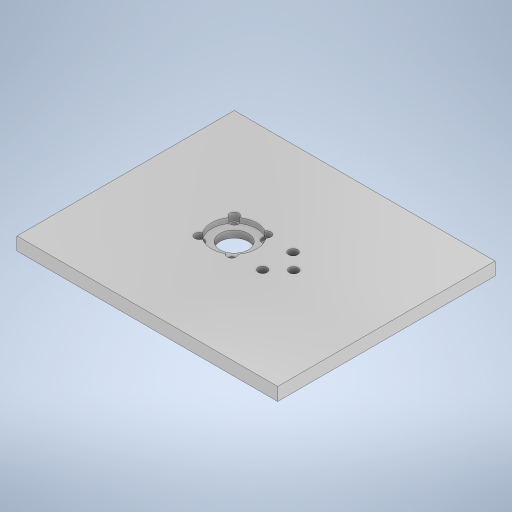
# Autodesk Inventor part: axis_1_top_frame
Saved by Autodesk Inventor 2024.1 (Build 281209000, 209)
## iProperties
Created: 2023-08-26
Part Number: axis_1_top_frame
Material: Aluminum 6061-AHC
Document SubType Name: Modeling
Designer: chanh
Density: 2.7 g/cm^3
Appearance: Aluminum - Dark
Author: chanh
Autodesk Inventor part; units mm, degrees
ref_plane "YZ Plane" through (0, 0, 0) normal (1, 0, 0) x (0, 1, 0)
ref_plane "XZ Plane" through (0, 0, 0) normal (0, 1, 0) x (-1, 0, 0)
ref_plane "XY Plane" through (0, 0, 0) normal (0, 0, 1) x (1, 0, 0)
sketch "Sketch1" plane through (0, 0, 0) normal (0, 1, 0) x (-1, 0, 0)
  line L0 (60, 50) -> (-60, 50)
  line L1 (-60, 50) -> (-60, -50)
  line L2 (-60, -50) -> (60, -50)
  line L3 (60, -50) -> (60, 50)
  line L4 (60, 50) -> (-60, -50) construction
  line L5 (-60, 50) -> (60, -50) construction
  point P0 (0, 0)
  dimension "d0" = 120
  dimension "d1" = 100
  constraints: 12 end point, 2 midpoint, 2 parallel, 1 horizontal, 1 perpendicular
  measures "d0" distance of L2.end L1.end
  measures "d1" distance of L1.end L0.end
extrude "Extrusion1" add sketch "Sketch1" along normal blind 6
sketch "Sketch3" plane through (0, 0, 0) normal (0, -1, 0) x (1, 0, 0)
  circle A0 centre (17.37, 0) radius 0.7835 projected
  circle A1 centre (10.07, 7) radius 0.7835 projected
  circle A2 centre (10.07, -7) radius 0.7835 projected
  circle A3 centre (-3.15, 8) radius 0.7835 projected
  circle A4 centre (-3.15, -8) radius 0.7835 projected
  line L0 (18.77, -6.07) -> (18.77, 6.07) projected
  line L1 (18.77, -6.07) -> (18.05, -6.07) projected
  arc A5 (18.05, -6.07) -> (16.05, -8.07) centre (18.05, -8.07) ccw projected
  line L2 (16.05, -8.07) -> (16.05, -8.79) projected
  line L3 (-16.05, -8.79) -> (16.05, -8.79) projected
  line L4 (-16.05, -8.79) -> (-16.05, -8.07) projected
  arc A6 (-16.05, -8.07) -> (-18.05, -6.07) centre (-18.05, -8.07) ccw projected
  line L5 (-18.05, -6.07) -> (-18.77, -6.07) projected
  line L6 (-18.77, 6.07) -> (-18.77, -6.07) projected
  line L7 (-18.77, 6.07) -> (-18.05, 6.07) projected
  arc A7 (-18.05, 6.07) -> (-16.05, 8.07) centre (-18.05, 8.07) ccw projected
  line L8 (-16.05, 8.07) -> (-16.05, 8.79) projected
  line L9 (16.05, 8.79) -> (-16.05, 8.79) projected
  line L10 (16.05, 8.79) -> (16.05, 8.07) projected
  arc A8 (16.05, 8.07) -> (18.05, 6.07) centre (18.05, 8.07) ccw projected
  line L11 (18.05, 6.07) -> (18.77, 6.07) projected
  circle A9 centre (-10.05, 0) radius 6.4 projected
  line L12 (19.09, 6.07) -> (19.09, -6.07)
  line L13 (16.05, -9.11) -> (-16.05, -9.11)
  line L14 (-19.09, -6.07) -> (-19.09, 6.07)
  line L15 (-16.05, 9.11) -> (16.05, 9.11)
  line L16 (16.05, 8.79) -> (16.05, 9.11)
  line L17 (18.77, 6.07) -> (19.09, 6.07)
  line L18 (18.77, -6.07) -> (19.09, -6.07)
  line L19 (16.05, -8.79) -> (16.05, -9.11)
  line L20 (-16.05, -8.79) -> (-16.05, -9.11)
  line L21 (-18.77, -6.07) -> (-19.09, -6.07)
  line L22 (-18.77, 6.07) -> (-19.09, 6.07)
  line L23 (-16.05, 8.79) -> (-16.05, 9.11)
  line L24 (16.15, 8.79) -> (16.15, 9.21)
  line L25 (16.15, 9.21) -> (-16.15, 9.21)
  line L26 (-16.15, 9.21) -> (-16.15, 8.79)
  line L27 (18.77, -6.17) -> (19.19, -6.17)
  line L28 (19.19, -6.17) -> (19.19, 6.17)
  line L29 (19.19, 6.17) -> (18.77, 6.17)
  line L30 (-16.15, -8.79) -> (-16.15, -9.21)
  line L31 (-16.15, -9.21) -> (16.15, -9.21)
  line L32 (16.15, -9.21) -> (16.15, -8.79)
  line L33 (-18.77, 6.17) -> (-19.19, 6.17)
  line L34 (-19.19, 6.17) -> (-19.19, -6.17)
  line L35 (-19.19, -6.17) -> (-18.77, -6.17)
  arc A10 (16.15, 8.07) -> (18.05, 6.17) centre (18.05, 8.07) ccw
  line L36 (16.15, 8.07) -> (16.15, 8.89)
  line L37 (-16.15, 8.89) -> (-16.15, 8.07)
  arc A11 (-18.05, 6.17) -> (-16.15, 8.07) centre (-18.05, 8.07) ccw
  line L38 (-18.05, 6.17) -> (-18.87, 6.17)
  line L39 (-18.87, -6.17) -> (-18.05, -6.17)
  arc A12 (-16.15, -8.07) -> (-18.05, -6.17) centre (-18.05, -8.07) ccw
  line L40 (-16.15, -8.07) -> (-16.15, -8.89)
  line L41 (16.15, -8.89) -> (16.15, -8.07)
  arc A13 (18.05, -6.17) -> (16.15, -8.07) centre (18.05, -8.07) ccw
  line L42 (18.05, -6.17) -> (18.87, -6.17)
  line L43 (18.87, 6.17) -> (18.05, 6.17)
  point P0 (0, 0)
  point P1 (-18.77, 6.17)
  point P2 (-18.87, -6.17)
  point P3 (11.8922, -6.17)
  dimension "d4" = 0.32
  dimension "d5" = 0.32
  dimension "d6" = 0.32
  dimension "d7" = 0.32
  dimension "d8" = 0.1
  dimension "d9" = 0.1
  dimension "d10" = 0.1
  dimension "d11" = 0.1
  dimension "d12" = 0.1
  constraints: 64 end point, 12 perpendicular, 8 point on circle, 4 centre point, 4 collinear, 2 point on line, 15 other
  measures "d4" distance between parallel lines of L0 L12
  measures "d5" distance between parallel lines of L13 L3
  measures "d6" distance between parallel lines of L15 L9
  measures "d7" distance between parallel lines of L6 L14
  measures "d8" distance between parallel lines of L15 L25
  measures "d9" distance between parallel lines of L12 L28
  measures "d10" distance between parallel lines of L13 L31
  measures "d11" distance between parallel lines of L14 L34
  measures "d12" radial gap between concentric circles of A8 A10
extrude "Extrusion2" cut sketch "Sketch3" against normal blind 0.5 contours A0 | A1 | A2 | A3 | A4 | L1 A5 L2 L3 L4 A6 L5 L6 L7 A7 L8 L9 L10 A8 L11 L0 | L0 L17 L12 L18 | L19 L13 L20 L3 | L9 L23 L15 L16 | L21 L14 L22 L6 | A9 | L36 A10 L43 L29 L28 L27 L42 A13 L41 L32 L31 L30 L40 A12 L39 L35 L34 L33 L38 A11 L37 L26 L25 L24
sketch "Sketch4" plane through (0, 0.5, 0) normal (0, -1, 0) x (1, 0, 0)
  circle A0 centre (-10.05, 0) radius 6.4 projected
  circle A1 centre (-10.05, 0) radius 6.5
  point P0 (0, 0)
  dimension "d15" = 0.1
  constraints: 1 centre point
  measures "d15" radial gap between concentric circles of A0 A1
sketch "Sketch5" plane through (0, 6, 0) normal (0, 1, 0) x (1, 0, 0)
  circle A0 centre (-10.05, 0) radius 1.2295 projected
  circle A1 centre (-10.05, 0) radius 10.4
  point P0 (0, 0)
  dimension "d16" = 20.8
  constraints: 1 centre point, 1 coincident
  measures "d16" diameter of A1
extrude "Extrusion3" cut sketch "Sketch5" against normal blind 2.3 contours A0 | A1
extrude "Extrusion4" cut sketch "Sketch4" against normal through all contours A0 | A1
hole "Hole1" at (-18.05, 6, -8.07) at (-18.05, 6, 8.07) at (-3.15, 6, 8) at (-3.15, 6, -8) at (10.07, 6, 7) at (17.37, 6, 0) at (10.07, 6, -7) direction (0, -1, 0) diameter 2.1 end through all
sketch "Sketch7" plane through (0, 0, 0) normal (0, -1, 0) x (1, 0, 0)
  arc A0 (16.15, 8.07) -> (18.05, 6.17) centre (18.05, 8.07) ccw projected
  arc A1 (18.05, -6.17) -> (16.15, -8.07) centre (18.05, -8.07) ccw projected
  circle A2 centre (18.05, 8.07) radius 0.85
  circle A3 centre (18.05, -8.07) radius 0.85
  point P0 (0, 0)
  dimension "d28" = 1.7
  constraints: 2 centre point, 2 coincident, 1 equal radius
  measures "d28" diameter of A2
extrude "Extrusion5" cut sketch "Sketch7" against normal blind 0.3
sketch "Sketch8" plane through (0, 6, 0) normal (0, 1, 0) x (1, 0, 0)
  arc A0 (-17.6502, -7.0991) -> (-17.0826, -7.6617) centre (-18.05, -8.07) ccw projected
  arc A1 (-17.0826, 7.6617) -> (-17.6502, 7.0991) centre (-18.05, 8.07) ccw projected
  arc A2 (-4.0689, -8.508) -> (-2.5125, -7.1657) centre (-3.15, -8) ccw projected
  arc A3 (-2.5125, 7.1657) -> (-4.0689, 8.508) centre (-3.15, 8) ccw projected
  circle A4 centre (10.07, -7) radius 1.05 projected
  circle A5 centre (17.37, 0) radius 1.05 projected
  circle A6 centre (10.07, 7) radius 1.05 projected
  circle A7 centre (-18.05, -8.07) radius 2.05
  circle A8 centre (-18.05, 8.07) radius 2.05
  circle A9 centre (-3.15, -8) radius 2.05
  circle A10 centre (-3.15, 8) radius 2.05
  circle A11 centre (10.07, 7) radius 2.05
  circle A12 centre (10.07, -7) radius 2.05
  circle A13 centre (17.37, 0) radius 2.05
  point P0 (0, 0)
  dimension "d31" = 4.1
  constraints: 7 centre point, 7 coincident, 6 equal radius
  measures "d31" diameter of A7
extrude "Extrusion6" cut sketch "Sketch8" against normal blind 3.5 contours A4 | A5 | A6 | A7 | A8 | A9 | A10 | A11 | A12 | A13
body "Solid1"
